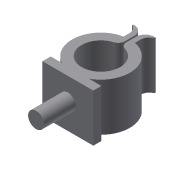
# Autodesk Inventor part: clip
Saved by Autodesk Inventor 2022 (Build 260148000, 148)
## iProperties
Created: 2006-05-17
Part Number: clip
Document SubType Name: Modeling
Designer: dchu
Density: 1 g/cm^3
Material: Generic
Appearance: Default
Author: dchu
Autodesk Inventor part; units mm, degrees
ref_plane "YZ Plane" through (0, 0, 0) normal (1, 0, 0) x (0, 1, 0)
ref_plane "XZ Plane" through (0, 0, 0) normal (0, 1, 0) x (-1, 0, 0)
ref_plane "XY Plane" through (0, 0, 0) normal (0, 0, 1) x (1, 0, 0)
sketch "Sketch1" plane through (0, 0, 0) normal (0, 0, 1) x (1, 0, 0)
  line L0 (-8.394, 13.4472) -> (-4.8398, 13.4472)
  line L1 (3.6697, 13.3964) -> (7.606, 13.3964)
  line L2 (-8.394, 13.4472) -> (-8.394, 10.8534)
  line L3 (-8.394, 10.8534) -> (7.606, 10.8534)
  line L4 (7.606, 10.8534) -> (7.606, 13.3964)
  arc A0 (-2.2893, 27.249) -> (1.0922, 27.249) centre (-0.5985, 21.4436) ccw
  line L5 (-2.341, 32.1588) -> (-2.341, 30.3259)
  arc A1 (-2.341, 32.1588) -> (-4.1098, 34.7456) centre (-5.117, 32.1588) ccw
  line L6 (-0.8485, 30.5374) -> (-0.8485, 32.1588)
  arc A2 (-0.8485, 32.1588) -> (-4.1098, 35.1104) centre (-3.8149, 32.1588) ccw
  line L7 (-4.1098, 35.1104) -> (-4.1098, 34.7456)
  arc A3 (3.6697, 13.3964) -> (1.1439, 30.3845) centre (-0.5985, 21.4436) ccw
  arc A4 (-2.341, 30.3259) -> (-4.8398, 13.4472) centre (-0.5985, 21.4436) ccw
  line L8 (-0.8485, 30.5374) -> (-0.8485, 29.1693)
  line L9 (-0.5985, 28.8881) -> (-0.5985, 21.4436) construction
  line L10 (1.1439, 32.1588) -> (1.1439, 30.3259)
  arc A5 (2.9127, 34.7456) -> (1.1439, 32.1588) centre (3.92, 32.1588) ccw
  line L11 (-0.3485, 30.5374) -> (-0.3485, 32.1588)
  arc A6 (2.9127, 35.1104) -> (-0.3485, 32.1588) centre (2.6178, 32.1588) ccw
  line L12 (2.9127, 35.1104) -> (2.9127, 34.7456)
  line L13 (-0.3485, 30.5374) -> (-0.3485, 29.1693)
  arc A7 (-2.2893, 27.249) -> (-0.8485, 29.1693) centre (-2.8485, 29.1693) ccw
  arc A8 (-0.3485, 29.1693) -> (1.0922, 27.249) centre (1.6515, 29.1693) ccw
  point P0 (-0.5985, 12.3345)
  dimension "d0" = 16
  dimension "d12" = 0.5
  dimension "d13" = 2
  constraints: 28 end point, 18 point on circle, 9 centre point, 8 symmetric about line, 6 tangent, 3 parallel, 2 perpendicular, 2 vertical alignment, 1 coincident, 1 equal radius, 1 point on line, 2 other
  measures "d0" distance of L0.start L1.end
  measures "d12" distance between parallel lines of L13 L8
  measures "d13" radius of A7
extrude "Extrusion1" add sketch "Sketch1" along normal mid plane 15
sketch "Sketch3" plane through (-8.394, 10.8534, 7.5) normal (0, -1, 0) x (1, 0, 0)
  line L0 (0, -15) -> (15.9999, -15) projected
  line L1 (15.9999, 0) -> (15.9999, -15) projected
  circle A0 centre (7.9999, -7) radius 2.5
  dimension "d14" = 5
  dimension "d15" = 8
  dimension "d16" = 8
  constraints: 1 centre point
  measures "d14" diameter of A0
  measures "d15" distance from line of L0 A0.centre
  measures "d16" distance from line of L1 A0.centre
extrude "Extrusion3" add sketch "Sketch3" along normal blind 10
body "Solid1"
